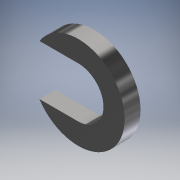
# Autodesk Inventor part: VS-006 (SPECIAL KEY)
Saved by Autodesk Inventor 2017 (Build 210142000, 142)
## iProperties
Created: 2016-12-05
Part Number: VS-006 (SPECIAL KEY)
Material: Steel, Carbon
Document SubType Name: Modeling
Designer: OCCC
Density: 7.85 g/cm^3
Appearance: Semi-Polished
Author: OCCC
Autodesk Inventor part; units mm, degrees
ref_plane "YZ Plane" through (0, 0, 0) normal (1, 0, 0) x (0, 1, 0)
ref_plane "XZ Plane" through (0, 0, 0) normal (0, 1, 0) x (-1, 0, 0)
ref_plane "XY Plane" through (0, 0, 0) normal (0, 0, 1) x (1, 0, 0)
sketch "Sketch1" plane through (0, 0, 0) normal (0, 0, 1) x (1, 0, 0)
  line L0 (-24.5181, 0) -> (28.4868, 0) construction
  arc A0 (-16.7905, -4.9609) -> (-16.7905, 4.9609) centre (-9.1281, 0) ccw
  arc A1 (-9.1281, -4.9609) -> (-9.1281, 4.9609) centre (-9.1281, 0) ccw
  line L1 (-9.1281, 4.9609) -> (-16.7905, 4.9609)
  line L2 (-9.1281, -4.9609) -> (-16.7905, -4.9609)
  point P0 (0, 0)
  dimension "d0" = 9.1281
  dimension "d1" = 9.9219
  constraints: 6 end point, 5 point on circle, 2 centre point, 2 point on line, 1 coincident, 1 horizontal, 1 parallel, 1 tangent, 1 other
  measures "d0" radius of A0
  measures "d1" distance between parallel lines of L2 L1
extrude "Extrusion1" add sketch "Sketch1" against normal blind 3.1369
body "Solid1"
